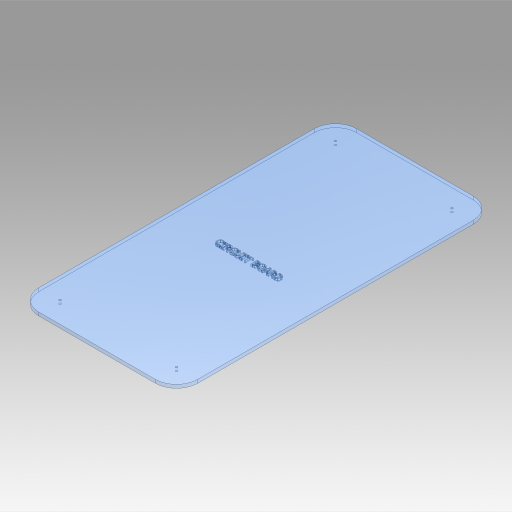
# Autodesk Inventor part: PCB
Saved by Autodesk Inventor 2023 (Build 270158000, 158)
## iProperties
Created: 2025-09-17
Part Number: PCB
Material: Generic
Document SubType Name: Modeling
Designer: NELLY NDUNG'U
Density: 1 g/cm^3
Appearance: Blue - Glazing
Author: NELLY NDUNG'U
Autodesk Inventor part; units mm, degrees
ref_plane "YZ Plane" through (0, 0, 0) normal (1, 0, 0) x (0, 1, 0)
ref_plane "XZ Plane" through (0, 0, 0) normal (0, 1, 0) x (-1, 0, 0)
ref_plane "XY Plane" through (0, 0, 0) normal (0, 0, 1) x (1, 0, 0)
sketch "Sketch1" plane through (0, 0, 0) normal (0, 1, 0) x (-1, 0, 0)
  line L0 (10, 0) -> (65, 0)
  line L1 (75, -10) -> (75, -140)
  line L2 (65, -150) -> (10, -150)
  line L3 (0, -140) -> (0, -10)
  arc A0 (65, -150) -> (75, -140) centre (65, -140) ccw
  arc A1 (75, -10) -> (65, 0) centre (65, -10) ccw
  arc A2 (0, -140) -> (10, -150) centre (10, -140) ccw
  arc A3 (10, 0) -> (0, -10) centre (10, -10) ccw
  circle A4 centre (65, -10) radius 0.5
  circle A5 centre (10, -10) radius 0.5
  circle A6 centre (65, -140) radius 0.5
  circle A7 centre (10, -140) radius 0.5
  point P0 (0, 0)
  point P1 (75, -150)
  point P2 (75, 0)
  point P3 (0, -150)
  dimension "d0" = 75
  dimension "d1" = 150
  dimension "d2" = 10
  dimension "d3" = 10
  dimension "d4" = 1
  dimension "d5" = 1
  dimension "d6" = 1
  dimension "d7" = 1
  constraints: 8 centre point, 8 end point, 8 point on circle, 8 point on line, 8 tangent, 4 coincident, 2 equal radius, 2 parallel, 1 horizontal, 1 perpendicular
  measures "d0" distance of point (75, -150) point (0, -150)
  measures "d1" distance of point (75, 0) point (75, -150)
  measures "d2" radius of A0
  measures "d3" radius of A1
  measures "d4" diameter of A4
  measures "d5" diameter of A5
  measures "d6" diameter of A6
  measures "d7" diameter of A7
extrude "Extrusion1" add sketch "Sketch1" along normal blind 1.6
sketch "Sketch2" plane through (0, 1.6, 0) normal (0, 1, 0) x (1, 0, 0)
  line L0 (-52.3194, 72.8493) -> (-21.6566, 72.8493) construction
  line L1 (-21.6566, 72.8493) -> (-21.6566, 69.6728) construction
  line L2 (-21.6566, 69.6728) -> (-52.3194, 69.6728) construction
  line L3 (-52.3194, 69.6728) -> (-52.3194, 72.8493) construction
  spline S0 degree 2 poles (-50.8201, 69.6827) (-51.1165, 69.6827) (-51.6179, 69.8828) (-51.8007, 70.0829) knots 0 0 0 1 2 2 2
  spline S1 degree 2 poles (-51.8007, 70.0829) (-51.9835, 70.2805) (-52.1836, 70.8733) (-52.1836, 71.2586) knots 0 0 0 1 2 2 2
  spline S2 degree 2 poles (-52.1836, 71.2586) (-52.1836, 71.6414) (-51.9884, 72.2095) (-51.8032, 72.4195) knots 0 0 0 1 2 2 2
  spline S3 degree 2 poles (-51.8032, 72.4195) (-51.6204, 72.6245) (-51.1215, 72.8394) (-50.8127, 72.8394) knots 0 0 0 1 2 2 2
  spline S4 degree 2 poles (-50.8127, 72.8394) (-50.6596, 72.8394) (-50.3903, 72.7949) (-50.2767, 72.7604) knots 0 0 0 1 2 2 2
  spline S5 degree 2 poles (-50.2767, 72.7604) (-50.1779, 72.7282) (-49.9729, 72.6369) (-49.8716, 72.5825) knots 0 0 0 1 2 2 2
  line L4 (-49.8716, 72.5825) -> (-49.8716, 72.0934)
  line L5 (-49.8716, 72.0934) -> (-49.9037, 72.0934)
  spline S6 degree 2 poles (-49.9037, 72.0934) (-49.9581, 72.1428) (-50.126, 72.2812) (-50.2471, 72.3479) knots 0 0 0 1 2 2 2
  spline S7 degree 2 poles (-50.2471, 72.3479) (-50.3632, 72.4121) (-50.6373, 72.4936) (-50.8152, 72.4936) knots 0 0 0 1 2 2 2
  spline S8 degree 2 poles (-50.8152, 72.4936) (-51.0103, 72.4936) (-51.3586, 72.333) (-51.4895, 72.1799) knots 0 0 0 1 2 2 2
  spline S9 degree 2 poles (-51.4895, 72.1799) (-51.6179, 72.0243) (-51.7612, 71.5525) (-51.7612, 71.2586) knots 0 0 0 1 2 2 2
  spline S10 degree 2 poles (-51.7612, 71.2586) (-51.7612, 70.9449) (-51.6105, 70.4929) (-51.4796, 70.3373) knots 0 0 0 1 2 2 2
  spline S11 degree 2 poles (-51.4796, 70.3373) (-51.3512, 70.1866) (-51.0078, 70.0335) (-50.8152, 70.0335) knots 0 0 0 1 2 2 2
  spline S12 degree 2 poles (-50.8152, 70.0335) (-50.6398, 70.0335) (-50.3409, 70.1199) (-50.2248, 70.1841) knots 0 0 0 1 2 2 2
  spline S13 degree 2 poles (-50.2248, 70.1841) (-50.1137, 70.2483) (-49.9482, 70.3817) (-49.9013, 70.4287) knots 0 0 0 1 2 2 2
  line L6 (-49.9013, 70.4287) -> (-49.8716, 70.4287)
  line L7 (-49.8716, 70.4287) -> (-49.8716, 69.9445)
  spline S14 degree 2 poles (-49.8716, 69.9445) (-49.9729, 69.8976) (-50.1507, 69.8112) (-50.2767, 69.7716) knots 0 0 0 1 2 2 2
  spline S15 degree 2 poles (-50.2767, 69.7716) (-50.4101, 69.7272) (-50.6373, 69.6827) (-50.8201, 69.6827) knots 0 0 0 1 2 2 2
  line L8 (-48.4316, 69.7371) -> (-49.6123, 69.7371)
  line L9 (-49.6123, 69.7371) -> (-49.6123, 70.0483)
  line L10 (-49.6123, 70.0483) -> (-49.2245, 70.0483)
  line L11 (-49.2245, 70.0483) -> (-49.2245, 72.4738)
  line L12 (-49.2245, 72.4738) -> (-49.6123, 72.4738)
  line L13 (-49.6123, 72.4738) -> (-49.6123, 72.7851)
  line L14 (-49.6123, 72.7851) -> (-48.4316, 72.7851)
  line L15 (-48.4316, 72.7851) -> (-48.4316, 72.4738)
  line L16 (-48.4316, 72.4738) -> (-48.8194, 72.4738)
  line L17 (-48.8194, 72.4738) -> (-48.8194, 70.0483)
  line L18 (-48.8194, 70.0483) -> (-48.4316, 70.0483)
  line L19 (-48.4316, 70.0483) -> (-48.4316, 69.7371)
  line L20 (-45.5713, 69.7371) -> (-46.0974, 69.7371)
  line L21 (-46.0974, 69.7371) -> (-47.0607, 70.9498)
  line L22 (-47.0607, 70.9498) -> (-47.5251, 70.9498)
  line L23 (-47.5251, 70.9498) -> (-47.5251, 69.7371)
  line L24 (-47.5251, 69.7371) -> (-47.9302, 69.7371)
  line L25 (-47.9302, 69.7371) -> (-47.9302, 72.7851)
  line L26 (-47.9302, 72.7851) -> (-47.1447, 72.7851)
  spline S16 degree 2 poles (-47.1447, 72.7851) (-46.8829, 72.7851) (-46.5297, 72.7282) (-46.3691, 72.6245) knots 0 0 0 1 2 2 2
  spline S17 degree 2 poles (-46.3691, 72.6245) (-46.2086, 72.5208) (-46.0233, 72.1972) (-46.0233, 71.9576) knots 0 0 0 1 2 2 2
  spline S18 degree 2 poles (-46.0233, 71.9576) (-46.0233, 71.6241) (-46.3642, 71.1721) (-46.6557, 71.0635) knots 0 0 0 1 2 2 2
  line L27 (-46.6557, 71.0635) -> (-45.5713, 69.7371)
  spline S19 degree 2 poles (-46.4457, 71.9255) (-46.4457, 72.0589) (-46.5396, 72.2639) (-46.6384, 72.3306) knots 0 0 0 1 2 2 2
  spline S20 degree 2 poles (-46.6384, 72.3306) (-46.7248, 72.3874) (-46.9545, 72.4343) (-47.1225, 72.4343) knots 0 0 0 1 2 2 2
  line L28 (-47.1225, 72.4343) -> (-47.5251, 72.4343)
  line L29 (-47.5251, 72.4343) -> (-47.5251, 71.2882)
  line L30 (-47.5251, 71.2882) -> (-47.1694, 71.2882)
  spline S21 degree 2 poles (-47.1694, 71.2882) (-46.9941, 71.2882) (-46.7149, 71.35) (-46.6186, 71.4463) knots 0 0 0 1 2 2 2
  spline S22 degree 2 poles (-46.6186, 71.4463) (-46.5297, 71.5303) (-46.4457, 71.7674) (-46.4457, 71.9255) knots 0 0 0 1 2 2 2
  spline S23 degree 2 poles (-44.1387, 69.6827) (-44.4351, 69.6827) (-44.9365, 69.8828) (-45.1193, 70.0829) knots 0 0 0 1 2 2 2
  spline S24 degree 2 poles (-45.1193, 70.0829) (-45.3021, 70.2805) (-45.5022, 70.8733) (-45.5022, 71.2586) knots 0 0 0 1 2 2 2
  spline S25 degree 2 poles (-45.5022, 71.2586) (-45.5022, 71.6414) (-45.307, 72.2095) (-45.1218, 72.4195) knots 0 0 0 1 2 2 2
  spline S26 degree 2 poles (-45.1218, 72.4195) (-44.939, 72.6245) (-44.4401, 72.8394) (-44.1313, 72.8394) knots 0 0 0 1 2 2 2
  spline S27 degree 2 poles (-44.1313, 72.8394) (-43.9782, 72.8394) (-43.7089, 72.7949) (-43.5953, 72.7604) knots 0 0 0 1 2 2 2
  spline S28 degree 2 poles (-43.5953, 72.7604) (-43.4965, 72.7282) (-43.2915, 72.6369) (-43.1902, 72.5825) knots 0 0 0 1 2 2 2
  line L31 (-43.1902, 72.5825) -> (-43.1902, 72.0934)
  line L32 (-43.1902, 72.0934) -> (-43.2223, 72.0934)
  spline S29 degree 2 poles (-43.2223, 72.0934) (-43.2767, 72.1428) (-43.4446, 72.2812) (-43.5657, 72.3479) knots 0 0 0 1 2 2 2
  spline S30 degree 2 poles (-43.5657, 72.3479) (-43.6818, 72.4121) (-43.9559, 72.4936) (-44.1338, 72.4936) knots 0 0 0 1 2 2 2
  spline S31 degree 2 poles (-44.1338, 72.4936) (-44.3289, 72.4936) (-44.6772, 72.333) (-44.8081, 72.1799) knots 0 0 0 1 2 2 2
  spline S32 degree 2 poles (-44.8081, 72.1799) (-44.9365, 72.0243) (-45.0798, 71.5525) (-45.0798, 71.2586) knots 0 0 0 1 2 2 2
  spline S33 degree 2 poles (-45.0798, 71.2586) (-45.0798, 70.9449) (-44.9291, 70.4929) (-44.7982, 70.3373) knots 0 0 0 1 2 2 2
  spline S34 degree 2 poles (-44.7982, 70.3373) (-44.6698, 70.1866) (-44.3264, 70.0335) (-44.1338, 70.0335) knots 0 0 0 1 2 2 2
  spline S35 degree 2 poles (-44.1338, 70.0335) (-43.9584, 70.0335) (-43.6595, 70.1199) (-43.5434, 70.1841) knots 0 0 0 1 2 2 2
  spline S36 degree 2 poles (-43.5434, 70.1841) (-43.4323, 70.2483) (-43.2668, 70.3817) (-43.2199, 70.4287) knots 0 0 0 1 2 2 2
  line L33 (-43.2199, 70.4287) -> (-43.1902, 70.4287)
  line L34 (-43.1902, 70.4287) -> (-43.1902, 69.9445)
  spline S37 degree 2 poles (-43.1902, 69.9445) (-43.2915, 69.8976) (-43.4693, 69.8112) (-43.5953, 69.7716) knots 0 0 0 1 2 2 2
  spline S38 degree 2 poles (-43.5953, 69.7716) (-43.7287, 69.7272) (-43.9559, 69.6827) (-44.1387, 69.6827) knots 0 0 0 1 2 2 2
  spline S39 degree 2 poles (-41.7477, 69.6728) (-42.017, 69.6728) (-42.4171, 69.8136) (-42.5579, 69.9544) knots 0 0 0 1 2 2 2
  spline S40 degree 2 poles (-42.5579, 69.9544) (-42.7185, 70.1125) (-42.8494, 70.5571) (-42.8494, 70.8831) knots 0 0 0 1 2 2 2
  line L35 (-42.8494, 70.8831) -> (-42.8494, 72.7851)
  line L36 (-42.8494, 72.7851) -> (-42.4443, 72.7851)
  line L37 (-42.4443, 72.7851) -> (-42.4443, 70.8831)
  spline S41 degree 2 poles (-42.4443, 70.8831) (-42.4443, 70.6707) (-42.3899, 70.3842) (-42.3134, 70.2681) knots 0 0 0 1 2 2 2
  spline S42 degree 2 poles (-42.3134, 70.2681) (-42.2319, 70.1446) (-41.9503, 70.0186) (-41.7477, 70.0186) knots 0 0 0 1 2 2 2
  spline S43 degree 2 poles (-41.7477, 70.0186) (-41.5575, 70.0186) (-41.2611, 70.1446) (-41.1796, 70.2681) knots 0 0 0 1 2 2 2
  spline S44 degree 2 poles (-41.1796, 70.2681) (-41.1031, 70.3842) (-41.0487, 70.6682) (-41.0487, 70.8733) knots 0 0 0 1 2 2 2
  line L38 (-41.0487, 70.8733) -> (-41.0487, 72.7851)
  line L39 (-41.0487, 72.7851) -> (-40.6436, 72.7851)
  line L40 (-40.6436, 72.7851) -> (-40.6436, 70.8831)
  spline S45 degree 2 poles (-40.6436, 70.8831) (-40.6436, 70.5645) (-40.7721, 70.11) (-40.9351, 69.9544) knots 0 0 0 1 2 2 2
  spline S46 degree 2 poles (-40.9351, 69.9544) (-41.0808, 69.8112) (-41.4662, 69.6728) (-41.7477, 69.6728) knots 0 0 0 1 2 2 2
  line L41 (-39.0011, 69.7371) -> (-40.1818, 69.7371)
  line L42 (-40.1818, 69.7371) -> (-40.1818, 70.0483)
  line L43 (-40.1818, 70.0483) -> (-39.794, 70.0483)
  line L44 (-39.794, 70.0483) -> (-39.794, 72.4738)
  line L45 (-39.794, 72.4738) -> (-40.1818, 72.4738)
  line L46 (-40.1818, 72.4738) -> (-40.1818, 72.7851)
  line L47 (-40.1818, 72.7851) -> (-39.0011, 72.7851)
  line L48 (-39.0011, 72.7851) -> (-39.0011, 72.4738)
  line L49 (-39.0011, 72.4738) -> (-39.3889, 72.4738)
  line L50 (-39.3889, 72.4738) -> (-39.3889, 70.0483)
  line L51 (-39.3889, 70.0483) -> (-39.0011, 70.0483)
  line L52 (-39.0011, 70.0483) -> (-39.0011, 69.7371)
  line L53 (-37.7883, 69.7371) -> (-37.7883, 72.4244)
  line L54 (-37.7883, 72.4244) -> (-38.8109, 72.4244)
  line L55 (-38.8109, 72.4244) -> (-38.8109, 72.7851)
  line L56 (-38.8109, 72.7851) -> (-36.3606, 72.7851)
  line L57 (-36.3606, 72.7851) -> (-36.3606, 72.4244)
  line L58 (-36.3606, 72.4244) -> (-37.3832, 72.4244)
  line L59 (-37.3832, 72.4244) -> (-37.3832, 69.7371)
  line L60 (-37.3832, 69.7371) -> (-37.7883, 69.7371)
  spline S47 degree 2 poles (-32.6754, 70.6732) (-32.6754, 70.4459) (-32.8483, 70.0977) (-32.9915, 69.9841) knots 0 0 0 1 2 2 2
  spline S48 degree 2 poles (-32.9915, 69.9841) (-33.1644, 69.8507) (-33.5572, 69.7371) (-33.8684, 69.7371) knots 0 0 0 1 2 2 2
  line L61 (-33.8684, 69.7371) -> (-34.7428, 69.7371)
  line L62 (-34.7428, 69.7371) -> (-34.7428, 72.7851)
  line L63 (-34.7428, 72.7851) -> (-33.9351, 72.7851)
  spline S49 degree 2 poles (-33.9351, 72.7851) (-33.609, 72.7851) (-33.283, 72.7431) (-33.1348, 72.6616) knots 0 0 0 1 2 2 2
  spline S50 degree 2 poles (-33.1348, 72.6616) (-32.9693, 72.5751) (-32.8186, 72.291) (-32.8186, 72.0984) knots 0 0 0 1 2 2 2
  spline S51 degree 2 poles (-32.8186, 72.0984) (-32.8186, 71.8835) (-33.0459, 71.5426) (-33.2459, 71.4463) knots 0 0 0 1 2 2 2
  line L64 (-33.2459, 71.4463) -> (-33.2459, 71.4315)
  spline S52 degree 2 poles (-33.2459, 71.4315) (-32.9742, 71.3574) (-32.6754, 70.9646) (-32.6754, 70.6732) knots 0 0 0 1 2 2 2
  spline S53 degree 2 poles (-33.0977, 70.6559) (-33.0977, 70.8288) (-33.1965, 71.0511) (-33.3447, 71.1301) knots 0 0 0 1 2 2 2
  spline S54 degree 2 poles (-33.3447, 71.1301) (-33.4411, 71.1795) (-33.6683, 71.2092) (-33.8783, 71.2092) knots 0 0 0 1 2 2 2
  line L65 (-33.8783, 71.2092) -> (-34.3377, 71.2092)
  line L66 (-34.3377, 71.2092) -> (-34.3377, 70.0829)
  line L67 (-34.3377, 70.0829) -> (-34.0092, 70.0829)
  spline S55 degree 2 poles (-34.0092, 70.0829) (-33.7424, 70.0829) (-33.4361, 70.1323) (-33.3176, 70.2113) knots 0 0 0 1 2 2 2
  spline S56 degree 2 poles (-33.3176, 70.2113) (-33.204, 70.2928) (-33.0977, 70.4953) (-33.0977, 70.6559) knots 0 0 0 1 2 2 2
  spline S57 degree 2 poles (-33.241, 72.0416) (-33.241, 72.1503) (-33.3151, 72.3133) (-33.3966, 72.3602) knots 0 0 0 1 2 2 2
  spline S58 degree 2 poles (-33.3966, 72.3602) (-33.4954, 72.4145) (-33.735, 72.4392) (-33.9499, 72.4392) knots 0 0 0 1 2 2 2
  line L68 (-33.9499, 72.4392) -> (-34.3377, 72.4392)
  line L69 (-34.3377, 72.4392) -> (-34.3377, 71.5476)
  line L70 (-34.3377, 71.5476) -> (-33.8783, 71.5476)
  spline S59 degree 2 poles (-33.8783, 71.5476) (-33.6881, 71.5476) (-33.5078, 71.5871) (-33.4114, 71.6488) knots 0 0 0 1 2 2 2
  spline S60 degree 2 poles (-33.4114, 71.6488) (-33.3176, 71.7081) (-33.241, 71.8983) (-33.241, 72.0416) knots 0 0 0 1 2 2 2
  spline S61 degree 2 poles (-30.1164, 72.4368) (-29.9435, 72.2342) (-29.7509, 71.6414) (-29.7509, 71.2611) knots 0 0 0 1 2 2 2
  spline S62 degree 2 poles (-29.7509, 71.2611) (-29.7509, 70.8905) (-29.9386, 70.2903) (-30.1164, 70.0878) knots 0 0 0 1 2 2 2
  spline S63 degree 2 poles (-30.1164, 70.0878) (-30.3042, 69.8754) (-30.8006, 69.6728) (-31.0995, 69.6728) knots 0 0 0 1 2 2 2
  spline S64 degree 2 poles (-31.0995, 69.6728) (-31.4083, 69.6728) (-31.9023, 69.8828) (-32.0826, 70.0878) knots 0 0 0 1 2 2 2
  spline S65 degree 2 poles (-32.0826, 70.0878) (-32.2579, 70.2903) (-32.4457, 70.8856) (-32.4457, 71.2611) knots 0 0 0 1 2 2 2
  spline S66 degree 2 poles (-32.4457, 71.2611) (-32.4457, 71.6439) (-32.2555, 72.2268) (-32.0801, 72.4368) knots 0 0 0 1 2 2 2
  spline S67 degree 2 poles (-32.0801, 72.4368) (-31.9023, 72.6393) (-31.4058, 72.8493) (-31.0995, 72.8493) knots 0 0 0 1 2 2 2
  spline S68 degree 2 poles (-31.0995, 72.8493) (-30.7883, 72.8493) (-30.2893, 72.6319) (-30.1164, 72.4368) knots 0 0 0 1 2 2 2
  spline S69 degree 2 poles (-30.1732, 71.2611) (-30.1732, 71.5624) (-30.3042, 72.0292) (-30.4227, 72.1824) knots 0 0 0 1 2 2 2
  spline S70 degree 2 poles (-30.4227, 72.1824) (-30.5437, 72.3404) (-30.8846, 72.4985) (-31.097, 72.4985) knots 0 0 0 1 2 2 2
  spline S71 degree 2 poles (-31.097, 72.4985) (-31.3169, 72.4985) (-31.6478, 72.3454) (-31.7738, 72.1824) knots 0 0 0 1 2 2 2
  spline S72 degree 2 poles (-31.7738, 72.1824) (-31.8948, 72.0268) (-32.0233, 71.5575) (-32.0233, 71.2611) knots 0 0 0 1 2 2 2
  spline S73 degree 2 poles (-32.0233, 71.2611) (-32.0233, 70.6608) (-31.5194, 70.0236) (-31.097, 70.0236) knots 0 0 0 1 2 2 2
  spline S74 degree 2 poles (-31.097, 70.0236) (-30.6747, 70.0236) (-30.1732, 70.6608) (-30.1732, 71.2611) knots 0 0 0 1 2 2 2
  line L71 (-29.6348, 69.7371) -> (-28.6073, 72.7851)
  line L72 (-28.6073, 72.7851) -> (-28.1083, 72.7851)
  line L73 (-28.1083, 72.7851) -> (-27.0808, 69.7371)
  line L74 (-27.0808, 69.7371) -> (-27.5081, 69.7371)
  line L75 (-27.5081, 69.7371) -> (-27.7847, 70.5892)
  line L76 (-27.7847, 70.5892) -> (-28.9481, 70.5892)
  line L77 (-28.9481, 70.5892) -> (-29.2248, 69.7371)
  line L78 (-29.2248, 69.7371) -> (-29.6348, 69.7371)
  line L79 (-27.8959, 70.935) -> (-28.3677, 72.3701)
  line L80 (-28.3677, 72.3701) -> (-28.837, 70.935)
  line L81 (-28.837, 70.935) -> (-27.8959, 70.935)
  line L82 (-24.4329, 69.7371) -> (-24.959, 69.7371)
  line L83 (-24.959, 69.7371) -> (-25.9223, 70.9498)
  line L84 (-25.9223, 70.9498) -> (-26.3867, 70.9498)
  line L85 (-26.3867, 70.9498) -> (-26.3867, 69.7371)
  line L86 (-26.3867, 69.7371) -> (-26.7918, 69.7371)
  line L87 (-26.7918, 69.7371) -> (-26.7918, 72.7851)
  line L88 (-26.7918, 72.7851) -> (-26.0063, 72.7851)
  spline S75 degree 2 poles (-26.0063, 72.7851) (-25.7445, 72.7851) (-25.3913, 72.7282) (-25.2307, 72.6245) knots 0 0 0 1 2 2 2
  spline S76 degree 2 poles (-25.2307, 72.6245) (-25.0702, 72.5208) (-24.8849, 72.1972) (-24.8849, 71.9576) knots 0 0 0 1 2 2 2
  spline S77 degree 2 poles (-24.8849, 71.9576) (-24.8849, 71.6241) (-25.2258, 71.1721) (-25.5173, 71.0635) knots 0 0 0 1 2 2 2
  line L89 (-25.5173, 71.0635) -> (-24.4329, 69.7371)
  spline S78 degree 2 poles (-25.3073, 71.9255) (-25.3073, 72.0589) (-25.4012, 72.2639) (-25.5, 72.3306) knots 0 0 0 1 2 2 2
  spline S79 degree 2 poles (-25.5, 72.3306) (-25.5864, 72.3874) (-25.8161, 72.4343) (-25.9841, 72.4343) knots 0 0 0 1 2 2 2
  line L90 (-25.9841, 72.4343) -> (-26.3867, 72.4343)
  line L91 (-26.3867, 72.4343) -> (-26.3867, 71.2882)
  line L92 (-26.3867, 71.2882) -> (-26.031, 71.2882)
  spline S80 degree 2 poles (-26.031, 71.2882) (-25.8557, 71.2882) (-25.5765, 71.35) (-25.4802, 71.4463) knots 0 0 0 1 2 2 2
  spline S81 degree 2 poles (-25.4802, 71.4463) (-25.3913, 71.5303) (-25.3073, 71.7674) (-25.3073, 71.9255) knots 0 0 0 1 2 2 2
  spline S82 degree 2 poles (-21.7875, 71.2586) (-21.7875, 70.8411) (-22.1259, 70.1693) (-22.41, 69.9816) knots 0 0 0 1 2 2 2
  spline S83 degree 2 poles (-22.41, 69.9816) (-22.6422, 69.8359) (-23.1189, 69.7371) (-23.4894, 69.7371) knots 0 0 0 1 2 2 2
  line L93 (-23.4894, 69.7371) -> (-24.1909, 69.7371)
  line L94 (-24.1909, 69.7371) -> (-24.1909, 72.7851)
  line L95 (-24.1909, 72.7851) -> (-23.4968, 72.7851)
  spline S84 degree 2 poles (-23.4968, 72.7851) (-23.067, 72.7851) (-22.5779, 72.6566) (-22.405, 72.543) knots 0 0 0 1 2 2 2
  spline S85 degree 2 poles (-22.405, 72.543) (-22.1111, 72.3479) (-21.7875, 71.7032) (-21.7875, 71.2586) knots 0 0 0 1 2 2 2
  spline S86 degree 2 poles (-22.2099, 71.2635) (-22.2099, 71.6143) (-22.4421, 72.1107) (-22.6718, 72.2515) knots 0 0 0 1 2 2 2
  spline S87 degree 2 poles (-22.6718, 72.2515) (-22.8348, 72.3479) (-23.2029, 72.4343) (-23.477, 72.4343) knots 0 0 0 1 2 2 2
  line L96 (-23.477, 72.4343) -> (-23.7858, 72.4343)
  line L97 (-23.7858, 72.4343) -> (-23.7858, 70.0878)
  line L98 (-23.7858, 70.0878) -> (-23.477, 70.0878)
  spline S88 degree 2 poles (-23.477, 70.0878) (-23.2078, 70.0878) (-22.8002, 70.1742) (-22.6348, 70.2903) knots 0 0 0 1 2 2 2
  spline S89 degree 2 poles (-22.6348, 70.2903) (-22.4223, 70.4336) (-22.2099, 70.9078) (-22.2099, 71.2635) knots 0 0 0 1 2 2 2
  point P0 (0, 0)
  constraints: 2 other
emboss "Emboss1" sketch "Sketch2" operation cut depth 1 direction (0, -1, 0)
body "Solid1"
